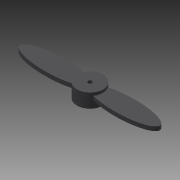
# Autodesk Inventor part: Baling2
Saved by Autodesk Inventor 2015 (Build 190159000, 159)
## iProperties
Created: 2015-02-02
Part Number: Baling2
Material: Generic
Document SubType Name: Modeling
Designer: Rafi Kurnia Putra
Density: 1 g/cm^3
Appearance: Gray
Mass: 1.85304 g
Surface Area: 18.4143 cm^2
Volume: 1.85304 cm^3
Author: Rafi Kurnia Putra
Autodesk Inventor part; units mm, degrees
ref_plane "YZ Plane" through (0, 0, 0) normal (1, 0, 0) x (0, 1, 0)
ref_plane "XZ Plane" through (0, 0, 0) normal (0, 1, 0) x (-1, 0, 0)
ref_plane "XY Plane" through (0, 0, 0) normal (0, 0, 1) x (1, 0, 0)
sketch "Sketch1" plane through (0, 0, 0) normal (0, 0, 1) x (1, 0, 0)
  circle A0 centre (0, 0) radius 6.5
  ellipse E0 centre (17.3675, 0) end of major axis (34.735, 0) minor radius 5.08
  line L0 (0, 30.8967) -> (0, 25.9123)
  ellipse E1 centre (-17.3675, 0) end of major axis (-34.735, 0) minor radius 5.08
  circle A1 centre (0, 0) radius 1
  circle A2 centre (0, 0) radius 1.6425
  circle A3 centre (0, 0) radius 2.3228
  dimension "d1" = 17.3675
  dimension "d2" = 5.08
  dimension "d0" = 13
  dimension "d7" = 2
  constraints: 4 centre point, 4 coincident, 2 end point, 2 vertical, 1 horizontal alignment, 1 symmetric about line, 4 other
  measures "d0" diameter of A0
  measures "d7" diameter of A1
extrude "Extrusion1" add sketch "Sketch1" along normal mid plane 6.93 contours A0 E0 A3 | E0 A3 E1 A0 | A0 E1 A3 E0 | E1 A3 A0 | A3 E0 A2 | E0 A2 E1 A3 | A3 E1 A2 E0 | E1 A2 A3 | A2 E0 A1 | E0 A1 E1 A2 | A2 E1 A1 E0 | E1 A1 A2 | A1 E0 | E0 E1 A1 | A1 E1 E0 | E1 A1
extrude "Extrusion2" add sketch "Sketch1" along normal blind 2 contours A0 E0 A3 | A0 E0 | E1 A3 A0 | A0 E1 | A3 E0 A2 | E1 A2 A3 | A2 E0 A1 | E1 A1 A2 | A1 E0 | E1 A1
extrude "Extrusion3" cut sketch "Sketch1" along normal through all both and the other way through all contours A1 E0 | E0 E1 A1 | A1 E1 E0 | E1 A1
extrude "Extrusion4" cut sketch "Sketch1" along normal blind 1 contours A2 E0 A1 | E0 A1 E1 A2 | A2 E1 A1 E0 | E1 A1 A2
extrude "Extrusion5" cut sketch "Sketch1" along normal blind 2 contours A3 E0 A2 | E0 A2 E1 A3 | A3 E1 A2 E0 | E1 A2 A3
sketch "Sketch2" plane through (0, 0, 2) normal (0, 0, 1) x (1, 0, 0)
  point P0 (0, 0)
body "Solid1"
